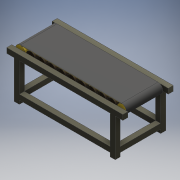
# Autodesk Inventor part: Traka
Saved by Autodesk Inventor 2016 (Build 200138000, 138)
## iProperties
Created: 2018-07-18
Part Number: Traka
Material: Generic
Document SubType Name: Modeling
Designer: semir
Density: 1 g/cm^3
Appearance: Default
Author: semir
Autodesk Inventor part; units mm, degrees
sketch "Sketch1" plane through (0, 0, 0) normal (0, 0, 1) x (1, 0, 0)
  line L0 (-200, 100) -> (200, -100) construction
  line L1 (200, 100) -> (-200, -100) construction
  line L2 (-200, 100) -> (-180, 100)
  line L3 (-180, 100) -> (-180, 80)
  line L4 (-180, 80) -> (-200, 80)
  line L5 (-200, 80) -> (-200, 100)
  line L6 (200, 100) -> (180, 100)
  line L7 (180, 100) -> (180, 80)
  line L8 (180, 80) -> (200, 80)
  line L9 (200, 80) -> (200, 100)
  line L10 (200, -100) -> (180, -100)
  line L11 (180, -100) -> (180, -80)
  line L12 (180, -80) -> (200, -80)
  line L13 (200, -80) -> (200, -100)
  line L14 (-200, -100) -> (-180, -100)
  line L15 (-180, -100) -> (-180, -80)
  line L16 (-180, -80) -> (-200, -80)
  line L17 (-200, -80) -> (-200, -100)
  line L18 (-200, 100) -> (-180, 100)
  line L19 (180, 100) -> (200, 100)
  line L20 (-200, -100) -> (-200, -80)
  line L21 (-200, 80) -> (-200, 100)
  line L22 (200, -100) -> (180, -100)
  line L23 (-180, -100) -> (-200, -100)
  line L24 (200, 100) -> (200, 80)
  line L25 (200, -80) -> (200, -100)
  point P0 (0, 0)
  dimension "d0" = 400
  dimension "d1" = 200
  dimension "d2" = 20
  dimension "d3" = 20
  dimension "d4" = 20
  dimension "d5" = 20
  dimension "d6" = 20
  dimension "d7" = 20
  dimension "d8" = 20
  dimension "d9" = 20
  constraints: 52 end point, 16 parallel, 8 perpendicular, 6 horizontal, 2 midpoint
  measures "d0" distance of L0.end L1.end
  measures "d1" distance of L1.start L0.end
  measures "d2" distance of L3.end L4.end
  measures "d3" distance of L2.end L3.end
  measures "d4" distance of L8.end L7.end
  measures "d5" distance of L7.end L6.end
  measures "d6" distance of L11.end L12.end
  measures "d7" distance of L10.end L11.end
  measures "d8" distance of L16.end L15.end
  measures "d9" distance of L15.end L14.end
extrude "Extrusion1" add sketch "Sketch1" along normal blind 150
sketch "Sketch2" plane through (-200, 80, 0) normal (-1, 0, 0) x (0, 0, 1)
  point P0 (0, -80)
sketch "Sketch3" plane through (-200, 80, 0) normal (-1, 0, 0) x (0, 0, 1)
  line L0 (0, 0) -> (150, 0) projected
  line L1 (0, -160) -> (150, -160) projected
  line L2 (34.9541, 0) -> (14.9541, 0)
  line L3 (14.9541, 0) -> (14.9541, -160)
  line L4 (14.9541, -160) -> (34.9541, -160)
  line L5 (34.9541, -160) -> (34.9541, 0)
  point P0 (0, -80)
  dimension "d12" = 20
  constraints: 8 end point, 2 parallel, 2 point on line, 1 horizontal, 1 perpendicular
  measures "d12" distance of L4.end L3.end
extrude "Extrusion2" add sketch "Sketch3" against normal blind 20
sketch "Sketch4" plane through (-200, -100, 0) normal (0, -1, 0) x (1, 0, 0)
  line L0 (20, 34.9541) -> (0, 34.9541) projected
  line L1 (0, 14.9541) -> (20, 14.9541) projected
  line L2 (380, 0) -> (380, 150) projected
  line L3 (20, 34.9541) -> (380, 34.9541)
  line L4 (380, 34.9541) -> (380, 14.9541)
  line L5 (380, 14.9541) -> (20, 14.9541)
  line L6 (20, 14.9541) -> (20, 34.9541)
  point P0 (200, 0)
  constraints: 8 end point, 2 parallel, 1 horizontal, 1 perpendicular, 1 point on line
extrude "Extrusion3" add sketch "Sketch4" against normal blind 20
ref_plane "Work Plane1" through (180, 0, 0) normal (0, -1, 0) x (1, 0, 0)
mirror "Mirror1" about plane through (180, 0, 0) normal (0, -1, 0) of "Extrusion3"
ref_plane "Work Plane2" through (0, 80, 0) normal (-1, 0, 0) x (0, 0, 1)
mirror "Mirror2" about plane through (0, 80, 0) normal (-1, 0, 0) of "Extrusion2"
sketch "Sketch5" plane through (180, -100, 0) normal (0, -1, 0) x (1, 0, 0)
  line L0 (-380, 14.9541) -> (-360, 14.9541) projected
  line L1 (-360, 34.9541) -> (-380, 34.9541) projected
  line L2 (-360, 0) -> (-360, 14.9541) projected
  line L3 (-380, 0) -> (-360, 0) projected
  line L4 (-380, 150) -> (-360, 150) projected
  line L5 (-410, 150) -> (50, 150)
  line L6 (50, 150) -> (50, 170)
  line L7 (50, 170) -> (-410, 170)
  line L8 (-410, 170) -> (-410, 150)
  line L9 (-380, 0) -> (-380, 150) projected
  line L10 (20, 0) -> (20, 150) projected
  point P0 (-180, 0)
  dimension "d17" = 14.9541
  dimension "d20" = 460
  dimension "d21" = 20
  dimension "d22" = 30
  constraints: 8 end point, 2 parallel, 1 horizontal, 1 perpendicular
  measures "d17" distance of L2.start L0.end
  measures "d20" distance of L7.end L6.end
  measures "d21" distance of L6.end L5.end
  measures "d22" distance from line of L5.start L9
extrude "Extrusion4" add sketch "Sketch5" against normal blind 20 contours L5 L8 L7 L6 L4
mirror "Mirror3" about plane through (180, 0, 0) normal (0, -1, 0) of "Extrusion4"
sketch "Sketch6" plane through (-200, 80, 34.9541) normal (0, -1, 0) x (1, 0, 0)
  point P0 (200, -34.9541)
ref_plane "Work Plane3" through (-200, 72.5, 34.9541) normal (0, -1, 0) x (1, 0, 0)
sketch "Sketch7" plane through (-200, 72.5, 34.9541) normal (0, -1, 0) x (1, 0, 0)
  circle A0 centre (-2.9279, 124.2812) radius 17.5 projected
  circle A1 centre (-2.9279, 124.2812) radius 17.5
  point P0 (200, -34.9541)
  dimension "d27" = 35
  constraints: 1 centre point, 1 coincident
  measures "d27" diameter of A1
extrude "Extrusion5" add sketch "Sketch7" along normal blind 145
pattern_linear "Rectangular Pattern1" count 11 spacing 40 along (1, 0, 0) of "Extrusion5"
sketch "Sketch11" plane through (-200, 80, 34.9541) normal (0, -1, 0) x (1, 0, 0)
  circle A0 centre (-2.9279, 124.2812) radius 17.5 projected
  circle A1 centre (-2.9279, 124.2812) radius 2.5
  point P0 (200, -34.9541)
  dimension "d33" = 5
  constraints: 1 centre point, 1 coincident
  measures "d33" diameter of A1
extrude "Extrusion6" add sketch "Sketch11" along normal up to surface (160 mm away) contours A1
pattern_linear "Rectangular Pattern2" count 11 spacing 40 along (1, 0, 0) of "Extrusion6"
ref_plane "Work Plane5" through (-200, -72.5, 34.9541) normal (0, 1, 0) x (1, 0, 0)
sketch "Sketch20" plane through (-200, -72.5, 34.9541) normal (0, 1, 0) x (1, 0, 0)
  circle A0 centre (-2.9279, -124.2812) radius 2.5 projected
  arc A1 (-2.9279, -106.7812) -> (-2.9279, -141.7812) centre (-2.9279, -124.2812) ccw
  circle A2 centre (397.0721, -124.2812) radius 2.5 projected
  line L0 (-2.9279, -141.7812) -> (397.0721, -141.7812)
  line L1 (-2.9279, -106.7812) -> (397.0721, -106.7812)
  circle A3 centre (397.0721, -124.2812) radius 17.5 projected
  arc A4 (397.0721, -141.7812) -> (397.0721, -106.7812) centre (397.0721, -124.2812) ccw
  circle A5 centre (397.0721, -124.2812) radius 17.5 projected
  line L2 (397.0721, -143.7812) -> (-2.9279, -143.7812)
  arc A6 (-2.9279, -104.7812) -> (-2.9279, -143.7812) centre (-2.9279, -124.2812) ccw
  line L3 (-2.9279, -104.7812) -> (397.0721, -104.7812)
  arc A7 (397.0721, -143.7812) -> (397.0721, -104.7812) centre (397.0721, -124.2812) ccw
  point P0 (200, 34.9541)
  dimension "d68" = 35
  dimension "d69" = 2
  constraints: 8 end point, 8 point on circle, 4 centre point, 3 tangent, 2 coincident, 2 horizontal, 3 other
  measures "d68" diameter of A4
  measures "d69" distance between parallel lines of L0 L2
extrude "Extrusion7" add sketch "Sketch20" along normal blind 145 contours L2 A6 L3 A7
body "Solid1"
